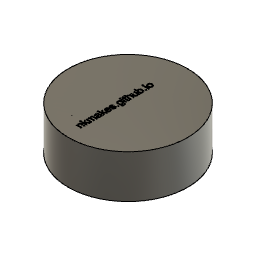
base_blank (Autodesk Fusion 360 design; units mm, degrees)
Autodesk Fusion 360 part; units mm, degrees
note: some values were not read from the file. Set by a fixed rule: which sketch regions a step uses.
sketch "Sketch1" plane through (0, 0, 0) normal (0, 1, 0) x (1, 0, 0)
  circle A0 centre (0, 0) radius 37.5
  circle A1 centre (0, 0) radius 38.7
  dimension "d1" = 75
  dimension "d2" = 1.2
  constraint coincident A0.centre A1.centre
  measures "d1" diameter of A0
extrude "Extrude1" add sketch "Sketch1" along normal blind 20
sketch "Sketch2" plane through (0, 20, 0) normal (0, 1, 0) x (-1, 0, 0)
  circle A0 centre (0, 0) radius 37.5
  circle A1 centre (0, 0) radius 38.7
  circle A2 centre (0, 0) radius 27.5
  line L0 (0, 0) -> (20, 0)
  line L1 (20, 0) -> (20, 31.7214)
  line L2 (20, 0) -> (20, -38.28)
  line L3 (0, 0) -> (-20, 0)
  line L4 (-20, 0) -> (-20, 43.7682)
  line L5 (-20, 0) -> (-20, -39.4022)
  dimension "d5" = 55
  dimension "d6" = 20
  dimension "d7" = 20
  constraint coincident A0.centre A1.centre
  constraint horizontal L0
  constraint coincident A0 L1.end
  constraint perpendicular L0 L1
  constraint perpendicular L0 L2
  constraint parallel L0 L3
  constraint perpendicular L3 L4
  constraint perpendicular L3 L5
  measures "d5" diameter of A2
  measures "d6" distance of A0.centre L0.end
  measures "d7" distance of A0.centre L3.end
extrude "Extrude2" add sketch "Sketch2" against normal blind 15 contours A0 A2 L1 L2 | A0 A2 L4 L5
sketch "Sketch3" plane through (0, 20, 0) normal (0, 1, 0) x (-1, 0, 0)
  line L0 (0, 0) -> (0, 25)
  line L1 (0, 25) -> (-14, 25)
  line L2 (0, 0) -> (0, -25)
  line L3 (0, -25) -> (14, -25)
  line L4 (-14, 25) -> (14, 25)
  line L5 (14, 25) -> (14, -25)
  line L6 (14, -25) -> (-14, -25)
  line L7 (-14, -25) -> (-14, 25)
  line L8 (14, 25) -> (14, 22.5)
  line L9 (14, 25) -> (11.5, 25)
  line L10 (14, 25) -> (11.5, 25)
  line L11 (11.5, 25) -> (11.5, 22.5)
  line L12 (11.5, 22.5) -> (14, 22.5)
  line L13 (14, 22.5) -> (14, 25)
  circle A0 centre (11.5, 22.5) radius 1.5
  circle A1 centre (-14, 25) radius 4
  circle A2 centre (14, 25) radius 4
  circle A3 centre (14, -25) radius 4
  circle A4 centre (-14, -25) radius 4
  circle A5 centre (0, 0) radius 27.5
  circle A6 centre (0, 0) radius 38.7
  dimension "d10" = 25
  dimension "d11" = 14
  dimension "d12" = 25
  dimension "d13" = 14
  dimension "d14" = 2.5
  dimension "d15" = 2.5
  dimension "d16" = 3
  dimension "d17" = 8
  dimension "d18" = 8
  dimension "d19" = 8
  dimension "d20" = 8
  constraint coincident L0.start L2.start
  constraint perpendicular L0 L1
  constraint perpendicular L2 L3
  constraint horizontal L4
  constraint vertical L5
  constraint horizontal L6
  constraint vertical L7
  constraint perpendicular L4 L8
  constraint perpendicular L5 L9
  constraint horizontal L10
  constraint vertical L11
  constraint horizontal L12
  constraint vertical L13
  constraint coincident L11.end L12.start
  constraint coincident L1.end L4.start
  constraint coincident L4.end L5.start
  constraint coincident L3.end L5.end
  constraint coincident L6.end L7.start
  constraint concentric A5 A6
  measures "d10" distance of L0.start L0.end
  measures "d11" distance of L0.end L1.end
  measures "d12" distance of L0.start L2.end
  measures "d13" distance of L2.end L3.end
  measures "d14" distance of L4.end L8.end
  measures "d15" distance of L4.end L9.end
  measures "d16" diameter of A0
  measures "d17" diameter of A1
  measures "d18" diameter of A2
  measures "d19" diameter of A3
  measures "d20" diameter of A4
extrude "Extrude3" add sketch "Sketch3" against normal blind 8 contours L1 L4 A1 A5 | L4 A2 A5 | L3 L6 A3 A5 | L6 A4 A5 | L1 L4 L7 A1 A5 | L7 A1 A5 | L4 L5 L8 L9 L10 L13 A2 A5 | L3 L5 L6 A3 A5 | L5 A3 A5 | L6 L7 A4 A5 | L7 A4 A5 | L5 L8 L13 A2 A5 | A6 picked at (-12.3161, 26.0387) picked at (12.3215, -26.043) picked at (-12.3161, -26.0387)
extrude "Extrude4" add sketch "Sketch3" against normal blind 5 contours L1 L4 L7 A1 A5 | L4 L11 A0 A2 A5 | L3 L5 L6 A3 A5 | L6 L7 A4 A5 | L1 L4 L7 A5 | L11 L12 A0 A2 | L3 L5 L6 A5 | L6 L7 A5 | L4 L5 L8 L9 L10 L11 L13 A5 | L5 L8 L11 L12 L13 A0 A5 | L11 L12 A0 | L5 L12 A0 A2 picked at (-13.1687, 23.0579) picked at (13.1687, -23.0579) picked at (-13.1687, -23.0579)
sketch "Sketch4" plane through (0, 12, 0) normal (0, -1, 0) x (1, 0, 0)
  line L0 (20, 18.8746) -> (20, 31.7214)
  arc A0 (20, 31.7214) -> (-20, 31.7214) centre (0, 0) ccw
  line L1 (-20, 31.7214) -> (-20, 18.8746)
  arc A1 (-16.5778, 21.9414) -> (-20, 18.8746) centre (0, 0) ccw
  arc A2 (-16.5778, 21.9414) -> (-14, 21) centre (-14, 25) ccw
  line L2 (-14, 21) -> (-14, 25)
  line L3 (-14, 25) -> (-10, 25)
  arc A3 (-10, 25) -> (-10.0452, 25.5997) centre (-14, 25) ccw
  arc A4 (10.0452, 25.5997) -> (-10.0452, 25.5997) centre (0, 0) ccw
  arc A5 (10.0452, 25.5997) -> (10, 25) centre (14, 25) ccw
  line L4 (10, 25) -> (14, 25)
  line L5 (14, 25) -> (14, 21)
  arc A6 (14, 21) -> (16.5778, 21.9414) centre (14, 25) ccw
  arc A7 (20, 18.8746) -> (16.5778, 21.9414) centre (0, 0) ccw
sketch "Sketch5" plane through (0, 12, 0) normal (0, -1, 0) x (1, 0, 0)
  line L0 (20, 18.8746) -> (20, 31.7214)
  arc A0 (20, 31.7214) -> (-20, 31.7214) centre (0, 0) ccw
  line L1 (-20, 31.7214) -> (-20, 18.8746)
  arc A1 (-16.5778, 21.9414) -> (-20, 18.8746) centre (0, 0) ccw
  arc A2 (-16.5778, 21.9414) -> (-14, 21) centre (-14, 25) ccw
  line L2 (-14, 21) -> (-14, 25)
  line L3 (-14, 25) -> (-10, 25)
  arc A3 (-10, 25) -> (-10.0452, 25.5997) centre (-14, 25) ccw
  arc A4 (10.0452, 25.5997) -> (-10.0452, 25.5997) centre (0, 0) ccw
  arc A5 (10.0452, 25.5997) -> (10, 25) centre (14, 25) ccw
  line L4 (10, 25) -> (14, 25)
  line L5 (14, 25) -> (14, 21)
  arc A6 (14, 21) -> (16.5778, 21.9414) centre (14, 25) ccw
  arc A7 (20, 18.8746) -> (16.5778, 21.9414) centre (0, 0) ccw
  line L6 (0, 0) -> (8, 0)
  line L7 (8, 0) -> (8, 53.7333)
  line L8 (8, 53.7333) -> (8, -45.4648)
  line L9 (0, 0) -> (-8, 0)
  line L10 (-8, 0) -> (-8, 52.3801)
  line L11 (-8, 52.3801) -> (-8, -45.2715)
  line L12 (-8, 48.2896) -> (8, 48.2896)
  line L13 (8, 48.2896) -> (8, -45.4648)
  line L14 (8, -45.4648) -> (-8, -45.4648)
  line L15 (-8, -45.4648) -> (-8, 48.2896)
  dimension "d25" = 8
  dimension "d26" = 8
  constraint coincident A0.centre A1.centre
  constraint horizontal L6
  constraint perpendicular L6 L7
  constraint perpendicular L6 L8
  constraint parallel L6 L9
  constraint perpendicular L9 L10
  constraint perpendicular L9 L11
  constraint horizontal L12
  constraint vertical L13
  constraint horizontal L14
  constraint vertical L15
  constraint coincident L10 L12.start
  measures "d25" distance of A0.centre L6.end
  measures "d26" distance of A0.centre L9.end
extrude "Extrude5" cut sketch "Sketch5" against normal blind 127.625 contours A0 A4 L7 L8 L10 L11 L13 L15
sketch "Sketch6" plane through (0, 12, 0) normal (0, -1, 0) x (1, 0, 0)
  line L0 (20, -31.7214) -> (20, -18.8746)
  arc A0 (16.5778, -21.9414) -> (20, -18.8746) centre (0, 0) ccw
  arc A1 (16.5778, -21.9414) -> (14, -21) centre (14, -25) ccw
  line L1 (14, -21) -> (14, -25)
  line L2 (14, -25) -> (10, -25)
  arc A2 (10, -25) -> (10.0452, -25.5997) centre (14, -25) ccw
  arc A3 (-10.0452, -25.5997) -> (10.0452, -25.5997) centre (0, 0) ccw
  arc A4 (-10.0452, -25.5997) -> (-10, -25) centre (-14, -25) ccw
  line L3 (-10, -25) -> (-14, -25)
  line L4 (-14, -25) -> (-14, -21)
  arc A5 (-14, -21) -> (-16.5778, -21.9414) centre (-14, -25) ccw
  arc A6 (-20, -18.8746) -> (-16.5778, -21.9414) centre (0, 0) ccw
  line L5 (-20, -18.8746) -> (-20, -31.7214)
  arc A7 (-20, -31.7214) -> (20, -31.7214) centre (0, 0) ccw
  line L6 (0, 0) -> (-8, 0)
  line L7 (0, 0) -> (8, 0)
  line L8 (8, 0) -> (8, -54.1754)
  line L9 (-8, 0) -> (-8, -51.6602)
  dimension "d29" = 8
  dimension "d30" = 8
  constraint coincident A0.centre A3.centre
  constraint horizontal L6
  constraint parallel L6 L7
  constraint perpendicular L7 L8
  constraint perpendicular L6 L9
  measures "d29" distance of A0.centre L6.end
  measures "d30" distance of A0.centre L7.end
extrude "Extrude6" cut sketch "Sketch6" against normal blind 79.742 contours A3 A7 L8 L9
sketch "Sketch7" plane through (0, 0, 0) normal (0, -1, 0) x (1, 0, 0)
  circle A0 centre (0, 0) radius 37.5
  circle A1 centre (0, 0) radius 38.7
  line L0 (0, 0) -> (0, -12)
  line L1 (0, 0) -> (0, 12)
  line L2 (0, 12) -> (-43.7804, 12)
  line L3 (-43.7804, 12) -> (-43.7804, -12)
  line L4 (-43.7804, -12) -> (0, -12)
  line L5 (0, -12) -> (0, 12)
  line L6 (-43.7804, -12) -> (35.5282, -12)
  line L7 (35.5282, -12) -> (35.5282, 12)
  line L8 (35.5282, 12) -> (-43.7804, 12)
  line L9 (-43.7804, 12) -> (-43.7804, -12)
  dimension "d33" = 12
  dimension "d34" = 12
  constraint coincident A0.centre A1.centre
  constraint vertical L0
  constraint parallel L0 L1
  constraint horizontal L2
  constraint vertical L3
  constraint horizontal L4
  constraint vertical L5
  constraint horizontal L6
  constraint vertical L7
  constraint horizontal L8
  constraint vertical L9
  constraint coincident A0 L7.end
  measures "d33" distance of A0.centre L0.end
  measures "d34" distance of A0.centre L1.end
extrude "Extrude7" cut sketch "Sketch7" against normal blind 62.051 contours A0 L7 | L0 L1 L5 L6 L7 L8 | A0 L0 L1 L2 L4 L5 L6 L8
sketch "Sketch8" plane through (0, 0, 0) normal (0, 0, 1) x (1, 0, 0)
  line L0 (0, 0) -> (0, 6.4234)
  circle A0 centre (0, 6.4234) radius 3.5
  line L1 (0, 6.4234) -> (0, 18.4581)
  circle A1 centre (0, 12.4408) radius 6
  dimension "d37" = 7
  dimension "d38" = 12
  constraint coincident L0.start origin
  constraint vertical L0
  constraint coincident L0.end A0.centre
  constraint parallel L0 L1
  constraint midpoint L1 A1.centre
  measures "d37" diameter of A0
  measures "d38" diameter of A1
extrude "Extrude8" cut sketch "Sketch8" against normal blind 57.186 contours A0 L1 A1 | A0 L1 A1 | A0 L1 A1 | A0 L1 A1
sketch "Sketch9" plane through (0, 20, 0) normal (0, 1, 0) x (-1, 0, 0)
  circle A0 centre (0, 0) radius 38.7
  line L0 (11.4564, 25) -> (11.5, 25)
  line L1 (11.5, 25) -> (11.5, 24.98)
  arc A1 (11.5, 24.98) -> (11.4564, 25) centre (0, 0) ccw
  line L2 (24.7437, 12) -> (35.5282, 12)
  arc A2 (35.5282, -12) -> (35.5282, 12) centre (0, 0) ccw
  line L3 (35.5282, -12) -> (24.7437, -12)
  arc A3 (16.5778, -21.9414) -> (24.7437, -12) centre (0, 0) ccw
  arc A4 (16.5778, -21.9414) -> (10.0452, -25.5997) centre (14, -25) ccw
  arc A5 (8, -26.3106) -> (10.0452, -25.5997) centre (0, 0) ccw
  line L4 (8, -26.3106) -> (8, -36.6367)
  arc A6 (-8, -36.6367) -> (8, -36.6367) centre (0, 0) ccw
  line L5 (-8, -36.6367) -> (-8, -26.3106)
  arc A7 (-10.0452, -25.5997) -> (-8, -26.3106) centre (0, 0) ccw
  arc A8 (-10.0452, -25.5997) -> (-16.5778, -21.9414) centre (-14, -25) ccw
  arc A9 (-24.7437, -12) -> (-16.5778, -21.9414) centre (0, 0) ccw
  line L6 (-24.7437, -12) -> (-35.5282, -12)
  arc A10 (-35.5282, 12) -> (-35.5282, -12) centre (0, 0) ccw
  line L7 (-35.5282, 12) -> (-24.7437, 12)
  arc A11 (-16.5778, 21.9414) -> (-24.7437, 12) centre (0, 0) ccw
  arc A12 (-16.5778, 21.9414) -> (-10.0452, 25.5997) centre (-14, 25) ccw
  arc A13 (-8, 26.3106) -> (-10.0452, 25.5997) centre (0, 0) ccw
  line L8 (-8, 26.3106) -> (-8, 36.6367)
  arc A14 (8, 36.6367) -> (-8, 36.6367) centre (0, 0) ccw
  line L9 (8, 36.6367) -> (8, 26.3106)
  arc A15 (10.0452, 25.5997) -> (8, 26.3106) centre (0, 0) ccw
  arc A16 (10.0452, 25.5997) -> (16.5778, 21.9414) centre (14, 25) ccw
  arc A17 (24.7437, 12) -> (16.5778, 21.9414) centre (0, 0) ccw
  circle A18 centre (0, 0) radius 38.7
  constraint coincident A0.centre A1.centre
extrude "Extrude9" add sketch "Sketch9" against normal blind 1.2 contours A0 A18 | L2 A2 L3 A3 A4 A5 L4 A6 L5 A7 A8 A9 L6 A10 L7 A11 A12 A13 L8 A14 L9 A15 A16 A17
fillet "Fillet1" radius 1.2 11 edges at (24.7437, 11.9, -12) (-24.7437, 11.9, -12) (-8, 15.4, -26.3106) (8, 15.4, -26.3106) (24.7437, 11.9, 12) (8, 15.4, 26.3106) (-8, 15.4, 26.3106) (-20, 8.5, 18.8746) (-24.7437, 11.9, 12) (20, 8.5, 18.8746) (-20, 8.5, -18.8746)
fillet "Fillet2" radius 1.6 4 edges at (-10.0452, 15.4, 25.5997) (10.0452, 15.4, -25.5997) (-10.0452, 15.4, -25.5997) (10.0452, 15.4, 25.5997)
fillet "Fillet3" radius 7 4 edges at (-16.5778, 15.4, 21.9414) (16.5778, 15.4, 21.9414) (-16.5778, 15.4, -21.9414) (16.5778, 15.4, -21.9414)
extrude "Extrude10" add 1 faces at (-37.847, 0, 0) along direction (0, -1, 0) blind 8
sketch "Sketch10" plane through (0, 12, 0) normal (0, -1, 0) x (1, 0, 0)
  arc A0 (8.8153, -26.0488) -> (8, -27.1855) centre (9.2, -27.1855) ccw
  line L0 (8, -27.1855) -> (8, -36.6367)
  arc A1 (8, -36.6367) -> (20, -31.7214) centre (0, 0) ccw
  line L1 (20, -31.7214) -> (20, -18.8743)
  arc A2 (14.3409, -21.0146) -> (20, -18.8743) centre (14.9375, -14.04) ccw
  arc A3 (14.3409, -21.0146) -> (14, -21) centre (14, -25) ccw
  line L2 (14, -21) -> (14, -25)
  line L3 (14, -25) -> (9.9403, -25)
  arc A4 (8.9434, -26.0051) -> (9.9403, -25) centre (8.4231, -24.4921) ccw
  arc A5 (8.8153, -26.0488) -> (8.9434, -26.0051) centre (0, 0) ccw
  line L4 (14, -25) -> (-14, -25)
  line L5 (-14, -25) -> (-14, 25)
  line L6 (-14, 25) -> (14, 25)
  line L7 (14, 25) -> (14, -25)
  line L8 (14, 25) -> (14.4, 25)
  line L9 (14.4, 25) -> (14.4, 25.4)
  line L10 (-14, -25) -> (-14.4, -25)
  line L11 (-14.4, -25) -> (-14.4, -25.4)
  line L12 (-14.4, -25.4) -> (14.4, -25.4)
  line L13 (14.4, -25.4) -> (14.4, 25.4)
  line L14 (14.4, 25.4) -> (-14.4, 25.4)
  line L15 (-14.4, 25.4) -> (-14.4, -25.4)
  line L16 (-14.4, 25.4) -> (-14.4, 25.8)
  line L17 (-14.4, 25.8) -> (14.4, 25.8)
  line L18 (14.4, 25.8) -> (14.4, 25.4)
  line L19 (14.4, 25.4) -> (-14.4, 25.4)
  line L20 (-14.4, 25.4) -> (-14.4, 25.8)
  line L21 (14.4, -25.4) -> (-14.4, -25.4)
  line L22 (-14.4, -25.4) -> (-14.4, -25.8)
  line L23 (-14.4, -25.8) -> (14.4, -25.8)
  line L24 (14.4, -25.8) -> (14.4, -25.4)
  point P0 (-14, 25)
  dimension "d48" = 0.4
  dimension "d49" = 0.4
  dimension "d50" = 0.4
  dimension "d51" = 0.4
  dimension "d54" = 0.4
  dimension "d55" = 0.4
  constraint horizontal L4
  constraint vertical L5
  constraint horizontal L6
  constraint vertical L7
  constraint coincident P0 L5.end
  constraint coincident A3.centre L2.end
  constraint horizontal L8
  constraint perpendicular L8 L9
  constraint perpendicular L5 L10
  constraint perpendicular L10 L11
  constraint horizontal L12
  constraint vertical L13
  constraint horizontal L14
  constraint vertical L15
  constraint perpendicular L14 L16
  constraint horizontal L17
  constraint vertical L18
  constraint horizontal L19
  constraint vertical L20
  constraint horizontal L21
  constraint vertical L22
  constraint horizontal L23
  constraint vertical L24
  measures "d48" distance of L6.end L8.end
  measures "d49" distance of L8.end L9.end
  measures "d50" distance of L4.end L10.end
  measures "d51" distance of L10.end L11.end
  measures "d54" distance of L14.end L16.end
  measures "d55" distance of L12.end L23.end
extrude "Extrude12" cut sketch "Sketch10" against normal blind 3 contours A4 L12 L21 L22 L23 | A4 L12 L21 L23 L24 | A4 L4 L10 L11 L12 L15 L21 | A2 A3 L2 L3 A4 L4 L7 L12 L13 L21 | A2 A3 L7 L8 L13 | L5 L6 L8 L9 L10 L13 L14 L15 L19 | L14 L16 L17 L18 L19 L20
extrude "Extrude11" cut sketch "Sketch10" against normal blind 3 contours A4 L4 L10 L11 L12 L15 L21 | A2 A3 L2 L3 A4 L4 L7 L12 L13 L21 | A2 A3 L7 L8 L13 | L5 L6 L8 L9 L10 L13 L14 L15 L19
sketch "Sketch11" plane through (0, 20, 0) normal (0, 1, 0) x (-1, 0, 0)
  circle A0 centre (0, 0) radius 38.7
  line L0 (11.4564, 25) -> (11.5, 25)
  line L1 (11.5, 25) -> (11.5, 24.98)
  arc A1 (11.5, 24.98) -> (11.4564, 25) centre (0, 0) ccw
  line L2 (0, 29.1855) -> (0, -18.5567) construction
  line L3 (0, -18.5567) -> (6, -18.5567) construction
  line L4 (6, -18.5567) -> (6, 29.1855) construction
  line L5 (6, 29.1855) -> (0, 29.1855) construction
  text T0 "nkmakes.github.io" font "Arial" height 6 align ink ink in box 0 x 0 at (0.02, 29.1755) x (0, -1) y (1, 0) spacing 1 height is em
  constraint perpendicular L2 L3
  constraint parallel L2 L4
  constraint parallel L3 L5
extrude "Extrude13" cut sketch "Sketch11" against normal blind 0.4 text T0
